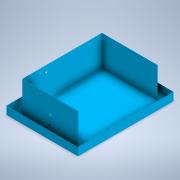
# Autodesk Inventor part: tub
Saved by Autodesk Inventor 2020 (Build 240168000, 168)
## iProperties
Created: 2020-04-13
Part Number: tub
Material: CFRP
Document SubType Name: Modeling
Designer: LENOVO
Density: 1.43 g/cm^3
Appearance: Carbon Fiber
Author: LENOVO
Autodesk Inventor part; units mm, degrees
ref_plane "YZ Plane" through (0, 0, 0) normal (1, 0, 0) x (0, 1, 0)
ref_plane "XZ Plane" through (0, 0, 0) normal (0, 1, 0) x (-1, 0, 0)
ref_plane "XY Plane" through (0, 0, 0) normal (0, 0, 1) x (1, 0, 0)
sketch "Sketch1" plane through (0, 0, 0) normal (0, 1, 0) x (-1, 0, 0)
  line L0 (345, 500) -> (-345, 500)
  line L1 (-345, -500) -> (345, -500)
  line L2 (350, -495) -> (350, 495)
  line L3 (350, 500) -> (-350, -500) construction
  line L4 (-350, 500) -> (350, -500) construction
  line L5 (347, 502) -> (-347, 502)
  line L6 (-347, -502) -> (347, -502)
  line L7 (352, -497) -> (352, 497)
  line L8 (352, 502) -> (-352, -502) construction
  line L9 (-352, 502) -> (352, -502) construction
  line L10 (445, 600) -> (-445, 600)
  line L11 (-450, 595) -> (-450, -595)
  line L12 (-445, -600) -> (445, -600)
  line L13 (450, -595) -> (450, 595)
  line L14 (450, 600) -> (-450, -600) construction
  line L15 (-450, 600) -> (450, -600) construction
  line L16 (447, 602) -> (-447, 602)
  line L17 (-452, 597) -> (-452, -597)
  line L18 (-447, -602) -> (447, -602)
  line L19 (452, -597) -> (452, 597)
  line L20 (452, 602) -> (-452, -602) construction
  line L21 (-452, 602) -> (452, -602) construction
  arc A0 (452, 597) -> (447, 602) centre (447, 597) ccw
  arc A1 (450, 595) -> (445, 600) centre (445, 595) ccw
  arc A2 (-445, 600) -> (-450, 595) centre (-445, 595) ccw
  arc A3 (-447, 602) -> (-452, 597) centre (-447, 597) ccw
  arc A4 (-450, -595) -> (-445, -600) centre (-445, -595) ccw
  arc A5 (-452, -597) -> (-447, -602) centre (-447, -597) ccw
  arc A6 (445, -600) -> (450, -595) centre (445, -595) ccw
  arc A7 (447, -602) -> (452, -597) centre (447, -597) ccw
  arc A8 (350, 495) -> (345, 500) centre (345, 495) ccw
  arc A9 (352, 497) -> (347, 502) centre (347, 497) ccw
  arc A10 (-345, 500) -> (-350, 495) centre (-345, 495) ccw
  arc A11 (-347, 502) -> (-352, 497) centre (-347, 497) ccw
  arc A12 (-352, -497) -> (-347, -502) centre (-347, -497) ccw
  arc A13 (-350, -495) -> (-345, -500) centre (-345, -495) ccw
  arc A14 (345, -500) -> (350, -495) centre (345, -495) ccw
  arc A15 (347, -502) -> (352, -497) centre (347, -497) ccw
  line L22 (-350, 495) -> (-352, 495)
  line L23 (-350, -495) -> (-352, -495)
  line L24 (-352, 497) -> (-352, 495)
  line L25 (-350, 466.6667) -> (-350, 466.1504)
  line L26 (-352, 469.3333) -> (-352, 468.8142)
  line L27 (-352, -495) -> (-352, -497)
  point P0 (0, 0)
  dimension "d0" = 700
  dimension "d1" = 1000
  dimension "d2" = 704
  dimension "d3" = 1004
  dimension "d4" = 900
  dimension "d5" = 1200
  dimension "d6" = 904
  dimension "d7" = 1204
  dimension "d8" = 5
  dimension "d9" = 5
  constraints: 56 end point, 36 tangent, 33 point on circle, 32 point on line, 16 centre point, 14 equal radius, 12 perpendicular, 10 parallel, 8 midpoint, 4 horizontal
  measures "d0" distance of L4.end L3.end
  measures "d1" distance of L3.end L4.start
  measures "d2" distance of L9.end L8.end
  measures "d3" distance of L8.end L9.start
  measures "d4" distance of L15.end L14.end
  measures "d5" distance of L14.end L15.start
  measures "d6" distance of L21.end L20.end
  measures "d7" distance of L20.end L21.start
  measures "d8" radius of A0
  measures "d9" radius of A2
extrude "Extrusion6" add sketch "Sketch1" along normal blind 2 contours A1 L13 A6 L12 A4 L11 A2 L10
extrude "Extrusion7" add sketch "Sketch1" along normal blind 392 contours L0 A10 L22 L24 A11 L5 A9 L7 A15 L6 A12 L27 L23 A13 L1 A14 L2 A8
extrude "Extrusion8" add sketch "Sketch1" along normal blind 100 contours A0 L19 A7 L18 A5 L17 A3 L16
sketch "Sketch2" plane through (-347, 2, 502) normal (0, 0, 1) x (1, 0, 0)
  line L0 (694, 0) -> (694, 390) projected
  line L1 (0, 390) -> (694, 390) projected
  point P0 (347, -2)
  point P1 (347, 200)
  dimension "d40" = 347
  dimension "d42" = 190
  measures "d40" distance from line of L0 point (347, 200)
  measures "d42" distance from line of L1 point (347, 200)
hole "Hole1" at (0, 202, 502) direction (0, 0, -1) diameter 5 depth 3 tip angle 118
sketch "Sketch3" plane through (-347, 2, 502) normal (0, 0, 1) x (1, 0, 0)
  line L0 (694, 0) -> (694, 390) projected
  line L1 (0, 390) -> (694, 390) projected
  point P0 (347, -2)
  point P1 (347, 170)
  dimension "d41" = 347
  dimension "d43" = 220
  measures "d41" distance from line of L0 point (347, 170)
  measures "d43" distance from line of L1 point (347, 170)
hole "Hole2" at (0, 172, 502) direction (0, 0, -1) diameter 30 depth 3 tip angle 118
sketch "Sketch4" plane through (-352, 2, 497) normal (-1, 0, 0) x (0, 0, 1)
  line L0 (0, 0) -> (0, 390) projected
  line L1 (-994, 390) -> (0, 390) projected
  point P0 (-497, -2)
  point P1 (-150, -20)
  point P2 (-300, 310)
  dimension "d58" = 300
  dimension "d59" = 150
  dimension "d60" = 80
  dimension "d61" = 410
  measures "d58" distance from line of point (-300, 310) L0
  measures "d59" distance from line of L0 point (-150, -20)
  measures "d60" distance from line of L1 point (-300, 310)
  measures "d61" distance from line of L1 point (-150, -20)
hole "Hole3" at (-352, -18, 347) at (-352, 312, 197) direction (1, 0, 0) diameter 20 depth 20
sketch "Sketch5" plane through (0, 2, 0) normal (0, 1, 0) x (1, 0, 0)
  line L0 (-352, -497) -> (-352, 497) projected
  point P0 (0, 0)
  point P1 (-392, -347)
  point P2 (-392, -197)
  dimension "d62" = 150
  dimension "d63" = 40
  dimension "d64" = 300
  dimension "d65" = 40
  measures "d62" vertical distance of L0.start point (-392, -347)
  measures "d63" distance from line of L0 point (-392, -347)
  measures "d64" vertical distance of L0.start point (-392, -197)
  measures "d65" distance from line of L0 point (-392, -197)
hole "Hole4" at (-392, 2, 347) at (-392, 2, 197) direction (0, -1, 0) diameter 20 depth 20
sketch "Sketch6" plane through (-347, 2, 502) normal (0, 0, 1) x (1, 0, 0)
  line L0 (694, 0) -> (0, 0) projected
  line L1 (0, 0) -> (0, 390) projected
  point P0 (347, -2)
  point P1 (340, 60)
  dimension "d73" = 60
  dimension "d74" = 340
  measures "d73" distance from line of L0 point (340, 60)
  measures "d74" distance from line of L1 point (340, 60)
hole "Hole5" at (-7, 62, 502) direction (0, 0, -1) diameter 25.4 depth 25.4 tip angle 118
sketch "Sketch7" plane through (0, 2, 0) normal (0, 1, 0) x (1, 0, 0)
  point P0 (0, 0)
  point P1 (-5, -535.191)
  point P2 (-345, -500)
  dimension "d82" = 340
  measures "d82" horizontal distance of point (-5, -535.191) point (-345, -500)
hole "Hole6" at (-5, 2, 535.191) direction (0, -1, 0) diameter 26 depth 26 tip angle 118
body "Solid2"
